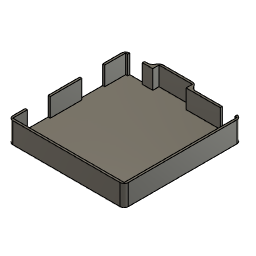
oled_boy_test_case v4 (Autodesk Fusion 360 design; units mm, degrees)
Autodesk Fusion 360 part; units mm, degrees
sketch "Sketch1" plane through (0, 0, 0) normal (0, 1, 0) x (1, 0, 0)
  line L0 (26.7, -27.05) -> (-26.7, -27.05)
  line L1 (-26.7, -27.05) -> (-26.7, 27.05)
  line L2 (-26.7, 27.05) -> (26.7, 27.05)
  line L3 (26.7, 27.05) -> (26.7, -27.05)
  line L4 (26.7, -27.05) -> (-26.7, 27.05) construction
  line L5 (-26.7, -27.05) -> (26.7, 27.05) construction
  line L6 (-27.7, -28.05) -> (-27.7, 28.05)
  line L7 (-27.7, 28.05) -> (27.7, 28.05)
  line L8 (27.7, 28.05) -> (27.7, -28.05)
  line L9 (27.7, -28.05) -> (-27.7, -28.05)
  dimension "d1" = 53.4
  dimension "d2" = 54.1
  dimension "d3" = -1
  constraint perpendicular L0 L1
  constraint parallel L0 L2
  constraint parallel L1 L3
  constraint horizontal L0
  constraint coincident L4 origin
  constraint coincident L5 origin
  measures "d1" distance of L1.end L2.end
  measures "d2" distance of L0.end L1.end
extrude "Extrude2" add sketch "Sketch1" along normal blind 1 contours L0 L1 L2 L3 makes body 1
extrude "Extrude1" add sketch "Sketch1" along normal blind 10 separate body makes body 2
sketch "Sketch2" plane through (-27.7, 0, 0) normal (-1, 0, 0) x (0, 0, 1)
  line L0 (-28.05, 0) -> (28.05, 0)
  line L1 (28.05, 0) -> (28.05, 10)
  line L2 (28.05, 10) -> (-28.05, 10)
  line L3 (-28.05, 10) -> (-28.05, 0)
  line L4 (-28.05, 5) -> (-6.05, 5)
  line L5 (-13, 0) -> (-13, 1)
  line L6 (-6.05, 1) -> (-17.05, 1)
  line L7 (-17.05, 1) -> (-17.05, 10)
  line L8 (-17.05, 10) -> (-6.05, 10)
  line L9 (-6.05, 10) -> (-6.05, 1)
  dimension "d8" = 22
  dimension "d9" = 11
  constraint midpoint L3 L4.start
  constraint perpendicular L3 L4
  constraint coincident L0 L5.start
  constraint perpendicular L0 L5
  constraint horizontal L6
  constraint vertical L7
  constraint horizontal L8
  constraint vertical L9
  constraint coincident L2 L7.end
  measures "d8" distance of L4.start L4.end
  measures "d9" distance of L6.start L6.end
extrude "Extrude3" cut sketch "Sketch2" against normal blind 16 contours L4 L6 L7 L9 | L2 L4 L7 L8 L9 bodies 2
sketch "Sketch3" plane through (0, 0, -28.05) normal (0, 0, -1) x (-1, 0, 0)
  line L0 (-27.7, 0) -> (27.7, 0)
  line L1 (27.7, 0) -> (27.7, 10)
  line L2 (27.7, 10) -> (-27.7, 10)
  line L3 (-27.7, 10) -> (-27.7, 0)
  line L4 (27.7, 5) -> (25.7, 5)
  line L5 (-27.7, 5) -> (-25.7, 5)
  line L6 (-23, 0) -> (-23, 1)
  line L7 (-25.7, 1) -> (-18.7, 1)
  line L8 (-18.7, 1) -> (-18.7, 10)
  line L9 (-18.7, 10) -> (-25.7, 10)
  line L10 (-25.7, 10) -> (-25.7, 1)
  line L11 (25.7, 1) -> (18.7, 1)
  line L12 (18.7, 1) -> (18.7, 10)
  line L13 (18.7, 10) -> (25.7, 10)
  line L14 (25.7, 10) -> (25.7, 1)
  dimension "d12" = 2
  dimension "d13" = 2
  dimension "d14" = 1
  dimension "d15" = 7
  dimension "d16" = 7
  constraint midpoint L1 L4.start
  constraint perpendicular L1 L4
  constraint midpoint L3 L5.start
  constraint perpendicular L3 L5
  constraint coincident L0 L6.start
  constraint perpendicular L0 L6
  constraint horizontal L7
  constraint vertical L8
  constraint horizontal L9
  constraint vertical L10
  constraint horizontal L11
  constraint vertical L12
  constraint horizontal L13
  constraint vertical L14
  constraint coincident L2 L12.end
  measures "d12" distance of L4.start L4.end
  measures "d13" distance of L5.start L5.end
  measures "d14" distance of L6.start L6.end
  measures "d15" distance of L7.start L7.end
  measures "d16" distance of L11.start L11.end
extrude "Extrude4" cut sketch "Sketch3" against normal blind 23 contours L2 L7 L8 L9 L10 | L2 L11 L12 L13 L14 bodies 2
sketch "Sketch4" plane through (0, 0, 0) normal (0, 1, 0) x (1, 0, 0)
  line L0 (-18.7, 28.05) -> (-13.7, 28.05)
  line L1 (-13.7, 28.05) -> (-13.7, 30.05)
  line L2 (-13.7, 30.05) -> (-7.7, 30.05)
  line L3 (-13.7, 28.05) -> (-13.7, 27.05)
  line L4 (-7.7, 27.05) -> (-13.7, 27.05)
  line L5 (-13.7, 27.05) -> (-13.7, 30.05)
  line L6 (-13.7, 30.05) -> (-7.7, 30.05)
  line L7 (-7.7, 30.05) -> (-7.7, 27.05)
  line L8 (-14.7, 26.05) -> (-14.7, 31.05)
  line L9 (-14.7, 31.05) -> (-6.7, 31.05)
  line L10 (-6.7, 31.05) -> (-6.7, 26.05)
  line L11 (-6.7, 26.05) -> (-14.7, 26.05)
  line L12 (-14.7, 28.05) -> (-13.7, 28.05)
  line L13 (-7.7, 28.05) -> (-6.7, 28.05)
  line L14 (-13.7, 28.05) -> (-7.7, 28.05)
  dimension "d19" = 5
  dimension "d20" = 2
  dimension "d21" = 6
  dimension "d22" = 1
  dimension "d23" = -1
  constraint horizontal L0
  constraint perpendicular L0 L1
  constraint perpendicular L1 L2
  constraint perpendicular L0 L3
  constraint horizontal L4
  constraint vertical L5
  constraint horizontal L6
  constraint vertical L7
  constraint coincident L2 L1.end
  constraint coincident L0 L12.start
  constraint coincident L8 L12.start
  constraint coincident L7 L13.start
  constraint coincident L10 L13.end
  constraint perpendicular L10 L13
  constraint perpendicular L7 L14
  measures "d19" distance of L0.start L0.end
  measures "d20" distance of L0.end L1.end
  measures "d21" distance of L1.end L2.end
  measures "d22" distance of L0.end L3.end
extrude "Extrude6" add sketch "Sketch4" along normal blind 10 contours L0 L1 L2 L5 L6 L7 L8 L9 L10 L12 L13 bodies 2
extrude "Extrude5" add sketch "Sketch4" along normal blind 1 contours L1 L2 L5 L6 L7 L14 bodies 2
sketch "Sketch5" plane through (0, 10, 0) normal (0, 1, 0) x (-1, 0, 0)
  line L0 (7.7, -28.05) -> (13.7, -28.05)
  line L1 (13.7, -28.05) -> (13.7, -30.05)
  line L2 (13.7, -30.05) -> (7.7, -30.05)
  line L3 (7.7, -30.05) -> (7.7, -28.05)
  line L4 (6.7, -28.05) -> (6.7, -31.05)
  line L5 (6.7, -31.05) -> (14.7, -31.05)
  line L6 (14.7, -31.05) -> (14.7, -28.05)
  line L7 (14.7, -28.05) -> (18.7, -28.05)
  line L8 (18.7, -28.05) -> (18.7, -27.05)
  line L9 (18.7, -27.05) -> (-18.7, -27.05)
  line L10 (-18.7, -27.05) -> (-18.7, -28.05)
  line L11 (-18.7, -28.05) -> (6.7, -28.05)
  line L12 (13.7, -28.05) -> (7.7, -28.05)
  line L13 (7.7, -28.05) -> (7.7, -27.05)
  line L14 (7.7, -27.05) -> (13.7, -27.05)
  line L15 (13.7, -27.05) -> (13.7, -28.05)
  constraint horizontal L12
  constraint vertical L13
  constraint horizontal L14
  constraint vertical L15
  constraint coincident L9 L13.end
  constraint coincident L0.end L1.start
extrude "Extrude7" cut sketch "Sketch5" against normal blind 9 contours L0 L9 L12 L13 L14 L15 bodies 2
sketch "Sketch6" plane through (-27.7, 0, 0) normal (-1, 0, 0) x (0, 0, 1)
  line L0 (-6.05, 10) -> (-6.05, 1)
  line L1 (-6.05, 1) -> (-17.05, 1)
  line L2 (-17.05, 1) -> (-17.05, 10)
  line L3 (-17.05, 10) -> (-28.05, 10)
  line L4 (-28.05, 10) -> (-28.05, 0)
  line L5 (-28.05, 0) -> (28.05, 0)
  line L6 (28.05, 0) -> (28.05, 10)
  line L7 (28.05, 10) -> (-6.05, 10)
  line L8 (28.05, 5) -> (20.05, 5)
  line L9 (21, 0) -> (21, 1)
  line L10 (20.05, 1) -> (9.05, 1)
  line L11 (9.05, 1) -> (9.05, 10.929)
  line L12 (9.05, 10.929) -> (20.05, 10.929)
  line L13 (20.05, 10.929) -> (20.05, 1)
  dimension "d30" = 8
  dimension "d31" = 11
  constraint midpoint L6 L8.start
  constraint perpendicular L6 L8
  constraint coincident L5 L9.start
  constraint perpendicular L5 L9
  constraint horizontal L10
  constraint vertical L11
  constraint horizontal L12
  constraint vertical L13
  measures "d30" distance of L8.start L8.end
  measures "d31" distance of L10.start L10.end
extrude "Extrude8" cut sketch "Sketch6" against normal blind 9 contours L7 L11 L12 L13 | L7 L10 L11 L13 bodies 2
combine "Combine1" operation add target body 1 tool bodies 2
sketch "Sketch7" plane through (0, 0, -27.05) normal (0, 0, 1) x (1, 0, 0)
  line L0 (-7.7, 1) -> (18.7, 1)
  line L1 (18.7, 1) -> (18.7, 10)
  line L2 (18.7, 10) -> (-7.7, 10)
  line L3 (-7.7, 10) -> (-7.7, 1)
  line L4 (-7.7, 10) -> (2.3, 10)
  line L5 (2.3, 10) -> (2.3, 1)
  line L6 (2.3, 1) -> (-7.7, 1)
  line L7 (-7.7, 1) -> (-7.7, 10)
  dimension "d34" = 10
  constraint horizontal L4
  constraint vertical L5
  constraint horizontal L6
  constraint vertical L7
  constraint coincident L2.end L3.start
  measures "d34" distance of L2.end L4.end
extrude "Extrude9" cut sketch "Sketch7" against normal blind 3 contours L0 L2 L3 L4 L5 L6 L7 bodies 1
sketch "Sketch8" plane through (0, 0, 0) normal (0, 1, 0) x (1, 0, 0)
extrude "Extrude10" add 1 faces at (-6.7, 3.6667, -30.7167) along direction (1, 0, 0) blind 9 on bodies 1 bodies 1
sketch "Sketch9" plane through (0, 0, -28.05) normal (0, 0, -1) x (-1, 0, 0)
  line L0 (-2.3, 0) -> (-2.3, 1)
  line L1 (-2.3, 1) -> (-2.3, 10)
  line L2 (-2.3, 10) -> (-18.7, 10)
  line L3 (-18.7, 10) -> (-18.7, 1)
  line L4 (-18.7, 1) -> (-25.7, 1)
  line L5 (-25.7, 1) -> (-25.7, 10)
  line L6 (-25.7, 10) -> (-27.7, 10)
  line L7 (-27.7, 10) -> (-27.7, 0)
  line L8 (-27.7, 0) -> (-2.3, 0)
  line L9 (-2.3, 10) -> (-3.3, 10)
  line L10 (-3.3, 10) -> (-3.3, 0)
  line L11 (-3.3, 0) -> (-2.3, 0)
  line L12 (-2.3, 0) -> (-2.3, 10)
  dimension "d39" = 1
  constraint horizontal L9
  constraint vertical L10
  constraint horizontal L11
  constraint vertical L12
  constraint coincident L8 L10.end
  constraint coincident L1.end L2.start
  measures "d39" distance of L1.end L9.end
extrude "Extrude11" add sketch "Sketch9" along normal blind 3 contours L0 L1 L2 L8 L9 L10 L11 L12 bodies 1
fillet "Fillet1" radius 2.5 4 edges at (-14.7, 5, -28.05) (-14.7, 5, -31.05) (3.3, 5, -28.05) (3.3, 5, -31.05) on bodies 1
fillet "Fillet2" radius 2 4 edges at (-27.7, 5, 28.05) (27.7, 5, 28.05) (-27.7, 5, -28.05) (27.7, 5, -28.05) on bodies 1
